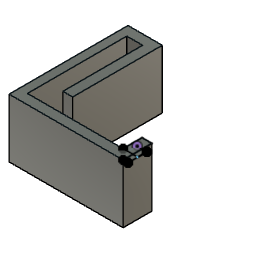
rail+proto-type-3x (Autodesk Fusion 360 design; units mm, degrees)
Autodesk Fusion 360 part; units mm, degrees
sketch "Sketch1" plane through (0, 0, 0) normal (0, 0, 1) x (1, 0, 0)
  line L0 (0, 0) -> (0, 20.32)
  line L1 (3, 20.32) -> (3, 1.5)
  line L2 (20.32, 3) -> (3, 3)
  line L3 (3, 3) -> (3, 1.5)
  line L4 (8.5, 2) -> (8.3025, 2)
  line L5 (20.32, 3) -> (20.32, 0)
  line L6 (0, 20.32) -> (3, 20.32)
  line L7 (22.32, 0) -> (22.32, 1)
  line L8 (19.558, -2) -> (0, -2)
  line L9 (-2, 19.558) -> (-2, -2)
  line L10 (-2, -2) -> (0, -2)
  line L11 (22.32, 0) -> (22.32, -2)
  line L12 (22.32, -2) -> (19.558, -2)
  line L13 (0, 22.32) -> (-2, 22.32)
  line L14 (-2, 22.32) -> (-2, 19.558)
  line L15 (0, 22.32) -> (1, 22.32)
  line L16 (5, 19.558) -> (5, 5)
  line L17 (5, 5) -> (19.558, 5)
  line L18 (1, 22.32) -> (5, 22.32)
  line L19 (5, 22.32) -> (5, 19.558)
  line L20 (19.558, 5) -> (10.5472, 5)
  line L21 (22.32, 1) -> (22.32, 5)
  line L22 (5, 5) -> (22.32, 5)
  line L23 (0, 0) -> (20.32, 0)
  dimension "d30" = 20.32
  dimension "d31" = 20.32
  dimension "d33" = 2
  dimension "d34" = 2
  dimension "d35" = 3
  dimension "d36" = 2
  dimension "d37" = 2
  dimension "d38" = 3
  constraint coincident L0.start L23.start
  constraint perpendicular L2 L3
  constraint perpendicular L1 L6
  constraint coincident L20 L21.end
  constraint perpendicular L20 L21
  constraint horizontal L17
  constraint horizontal L20
  constraint perpendicular L5 L23
  constraint perpendicular L0 L23
  constraint perpendicular L0 L6
  measures "d30" distance of L0.start L0.end
  measures "d31" distance of L5.end L0.start
  measures "d33" distance of L5 L7
  measures "d34" distance of L6 L15
  measures "d35" distance of L0.end L1.start
  measures "d36" distance of L1 L16
  measures "d37" distance of L2 L20
  measures "d38" distance of L2.start L5.end
sketch "Sketch2" plane through (0, 0, 0) normal (0, 0, 1) x (-1, 0, 0)
  line L0 (-8.5, 0) -> (0, 0)
  line L1 (0, 0) -> (0, -8.35)
  line L2 (0, -8.35) -> (-1, -8.35)
  line L3 (-1, -8.35) -> (-1, -1)
  line L4 (-1, -1) -> (-8.5, -1)
  line L5 (-9.5, -2) -> (-2, -2)
  line L6 (-2, -9.35) -> (1, -9.35)
  line L7 (1, -9.35) -> (1, -8.35)
  line L8 (-9.5, 0.9516) -> (-9.5, -2)
  line L9 (-3.5, -1) -> (-1, -1)
  line L10 (-1, -1) -> (-1, -4)
  line L11 (-1, -4) -> (-3.5, -4)
  line L12 (-3.5, -4) -> (-3.5, -1)
  line L13 (-3.5, -1) -> (-1, -1)
  line L14 (-1, -4) -> (-1, -1)
  line L15 (-3.5, -1) -> (-1, -1)
  line L16 (1, -8.35) -> (1, 0.9516)
  line L17 (1, 0.9516) -> (-9.5, 0.9516)
  line L18 (-1, -4) -> (-1, -8)
  line L19 (-3.5, -1) -> (-7.5, -1)
  line L20 (-1, -8) -> (-7.5024, -8)
  line L21 (-7.5024, -8) -> (-7.5, -1)
  dimension "d29" = 4
  constraint horizontal L9
  constraint vertical L10
  constraint horizontal L11
  constraint vertical L12
  constraint coincident L3 L10.end
  constraint coincident L4 L9.start
  constraint coincident L3 L18.end
  constraint perpendicular L2 L18
  constraint perpendicular L12 L19
  constraint perpendicular L18 L20
  measures "d29" distance of L9.start L19.end
extrude "Extrude3" add sketch "Sketch1" along normal blind 8
extrude "Extrude4" cut sketch "Sketch2" along normal blind 10
sketch "Sketch3" plane through (0, 0, 8) normal (0, 0, 1) x (-1, 0, 0)
  line L0 (-3, -8) -> (-5, -8)
  line L1 (-5, -8) -> (-5, -22.32)
  line L2 (-5, -22.32) -> (2, -22.32)
  line L3 (2, -22.32) -> (2, 2)
  line L4 (2, 2) -> (-22.32, 2)
  line L5 (-22.32, 2) -> (-22.32, -5)
  line L6 (-22.32, -5) -> (-7.5014, -5)
  line L7 (-7.5014, -5) -> (-7.5007, -3)
  line L8 (-7.5007, -3) -> (-20.32, -3)
  line L9 (-20.32, -3) -> (-20.32, 0)
  line L10 (-20.32, 0) -> (0, 0)
  line L11 (0, 0) -> (0, -20.32)
  line L12 (0, -20.32) -> (-3, -20.32)
  line L13 (-3, -20.32) -> (-3, -8)
  line L14 (-5, 0) -> (-5, 0)
  line L15 (-5, 0) -> (-5, -5.022)
  line L16 (-5, -5.022) -> (-5, -5.022)
  line L17 (-5, -5.022) -> (-5, 0)
  line L18 (-22.32, 2) -> (-5, 2)
  line L19 (-5, 2) -> (-5, 2)
  line L20 (-5, 2) -> (-22.32, 2)
  line L21 (-22.32, 2) -> (-22.32, 2)
  line L22 (-5, -5.022) -> (-22.32, -5.022)
  line L23 (-22.32, -5.022) -> (-22.32, -5)
  line L24 (-22.32, -5) -> (-5, -5)
  line L25 (-5, -5) -> (-5, -5.022)
  line L26 (-5, 2) -> (-5, 0)
  line L27 (-22.32, -1.8791) -> (-5, -1.8791)
  constraint vertical L15
  constraint vertical L17
  constraint coincident L10 L14.start
  constraint horizontal L18
  constraint horizontal L20
  constraint coincident L4 L18.end
  constraint coincident L4.end L5.start
  constraint horizontal L22
  constraint vertical L23
  constraint horizontal L24
  constraint vertical L25
  constraint coincident L5.end L6.start
  constraint coincident L5 L27.start
  constraint coincident L15 L27.end
  constraint perpendicular L15 L27
extrude "Extrude5" cut sketch "Sketch3" against normal blind 8 contours L7 L8 L9 L15 L17 L24 L27 | L5 L6 L7 L8 L9 L24 L27
extrude "Extrude6" add 1 faces at (-1.3333, 13.5467, 8) along direction (0, 0, 1) blind 4
sketch "Sketch4" plane through (0, 0, 12) normal (0, 0, 1) x (-1, 0, 0)
  line L0 (-20.32, 0) -> (0, 0)
  line L1 (-3, -20.32) -> (-3, -8)
  line L2 (-3, -8) -> (-5, -8)
  line L3 (-5, -8) -> (-5, -22.32)
  line L4 (-5, -22.32) -> (2, -22.32)
  line L5 (2, -22.32) -> (2, 2)
  line L6 (2, 2) -> (-22.32, 2)
  line L7 (0, 0) -> (0.25, 0)
  line L8 (0, -20.32) -> (0, 0)
  line L9 (0.25, 0) -> (0.25, -20.5)
  line L10 (0, -20.32) -> (0.25, -20.32)
  line L11 (-22.32, -1.8791) -> (-20.32, -1.8791)
  line L12 (-20.32, -1.8791) -> (-20.32, 0)
  line L13 (-22.32, 2) -> (-22.32, -1.8791)
  dimension "d44" = 0.25
  constraint coincident L0.end L7.start
  constraint parallel L0 L7
  constraint perpendicular L0 L8
  constraint perpendicular L7 L9
  constraint coincident L9 L10.end
  constraint perpendicular L9 L10
  measures "d44" distance of L0.end L7.end
extrude "Extrude7" cut sketch "Sketch4" against normal blind 12
extrude "Extrude8" add 1 faces at (4.3333, 8, 4) along direction (0, -1, 0) blind 4
sketch "Sketch5" plane through (0, 0, 12) normal (0, 0, 1) x (-1, 0, 0)
  line L0 (-20.32, 0) -> (0.25, 0)
  line L1 (0.25, 0) -> (0.25, -20.32)
  line L2 (0.25, -20.32) -> (-3, -20.32)
  line L3 (-3, -20.32) -> (-3, -4)
  line L4 (-3, -4) -> (-5, -4)
  line L5 (-5, -4) -> (-5, -22.32)
  line L6 (-5, -22.32) -> (2, -22.32)
  line L7 (2, -22.32) -> (2, 2)
  line L8 (2, 2) -> (-22.32, 2)
  line L9 (-22.32, 2) -> (-22.32, -1.8791)
  line L10 (-22.32, -1.8791) -> (-20.32, -1.8791)
  line L11 (-20.32, -1.8791) -> (-20.32, 0)
  line L12 (-21.32, -1.8791) -> (-20.32, -1.8791)
  line L13 (-19.32, -1.8791) -> (-19.32, 0)
  line L14 (-22.32, 0.0604) -> (-22.1613, 0)
  line L15 (-22.1613, 0) -> (-19.32, 0)
  line L16 (-22.32, -1.8791) -> (-22.32, 0.0604)
  line L17 (-21.32, -1.8791) -> (-21.32, 0)
  line L18 (-19.32, -1.8791) -> (-19.32, -3.8791)
  line L19 (-19.32, -3.8791) -> (-21.32, -3.8791)
  line L20 (-21.32, -1.8791) -> (-21.32, -3.8791)
  line L21 (-21.32, -1.8791) -> (-22.32, -1.8791)
  line L22 (-21.32, 0) -> (-21.32, 2)
  line L23 (-22.32, 2) -> (-22.32, -1.8791)
  line L24 (-21.32, -1.8791) -> (-22.32, -1.8791)
  line L25 (-21.32, 2) -> (-22.32, 2)
  dimension "d49" = 2
  dimension "d50" = 2
  constraint midpoint L10 L12.start
  constraint perpendicular L11 L12
  constraint coincident L0 L13.end
  constraint perpendicular L0 L13
  constraint midpoint L9 L14.start
  constraint perpendicular L13 L15
  constraint coincident L9.end L10.start
  constraint coincident L15 L17.end
  constraint perpendicular L15 L17
  constraint perpendicular L12 L18
  constraint perpendicular L18 L19
  constraint perpendicular L19 L20
  constraint coincident L8 L22.end
  constraint perpendicular L8 L22
  constraint coincident L8.end L9.start
  measures "d49" distance of L12.start L13.start
  measures "d50" distance of L13.start L18.end
extrude "Extrude9" cut sketch "Sketch5" against normal blind 12 contours L9 L10 L14 L15 L16 L17 L21 L23 L24 | L8 L9 L14 L15 L22 L23 L25
extrude "Extrude10" add sketch "Sketch5" against normal blind 12 contours L0 L10 L11 L12 L13 L15 L18 L19 L20
